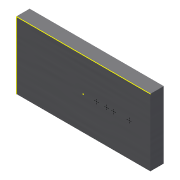
# Autodesk Inventor part: Placement
Saved by Autodesk Inventor 2022 Beta2 (Build 260130000, 130) ContinuousBuild 0
## iProperties
Created: 2009-02-24
Part Number: Placement
Document SubType Name: Modeling
Designer: User
Density: 1 g/cm^3
Material: Generic
Appearance: Light Gray
Author: User
Autodesk Inventor part; units mm, degrees
ref_plane "YZ Plane" through (0, 0, 0) normal (1, 0, 0) x (0, 1, 0)
ref_plane "XZ Plane" through (0, 0, 0) normal (0, 1, 0) x (-1, 0, 0)
ref_plane "XY Plane" through (0, 0, 0) normal (0, 0, 1) x (1, 0, 0)
sketch "Sketch1" plane through (0, 0, 0) normal (0, 0, 1) x (1, 0, 0)
  line L0 (-127, 63.5) -> (127, 63.5)
  line L1 (127, 63.5) -> (127, -63.5)
  line L2 (127, -63.5) -> (-127, -63.5)
  line L3 (-127, -63.5) -> (-127, 63.5)
  line L4 (-127, 63.5) -> (127, -63.5) construction
  point P0 (0, 0)
  point P1 (0, 0)
  dimension "BLlength" = 254
  dimension "BLwidth" = 127
  constraints: 10 end point, 2 parallel, 1 coincident, 1 horizontal, 1 midpoint, 1 perpendicular
  measures "BLlength" distance of L0.start L0.end
  measures "BLwidth" distance of L2.end L0.start
extrude "Extrusion1" add sketch "Sketch1" against normal blind 25.4
sketch "Sketch2" plane through (0, 0, 0) normal (0, 0, 1) x (1, 0, 0)
  line L0 (-127, 63.5) -> (127, 63.5) projected
  line L1 (-127, -63.5) -> (-127, 63.5) projected
  point P0 (0, 0)
  point P1 (25.2505, 0)
  point P2 (44.2485, 0)
  point P3 (57.731, 0)
  point P4 (86.8409, 0)
  constraints: 4 horizontal alignment
body "Solid1"
